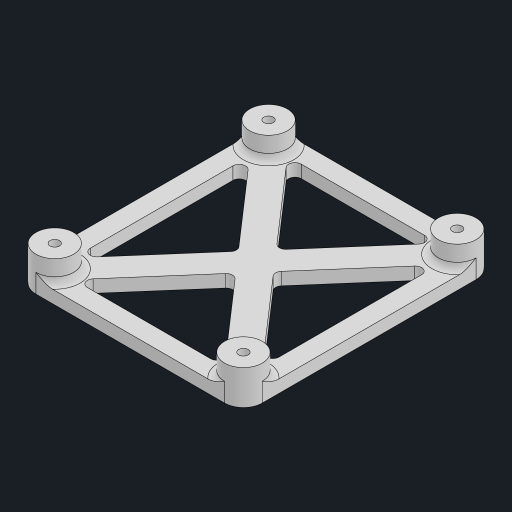
# Autodesk Inventor part: kibanHolder
Saved by Autodesk Inventor 2023 (Build 270158000, 158)
## iProperties
Created: 2022-07-14
Part Number: kibanHolder
Material: 一般
Document SubType Name: Modeling
Designer: legot
Density: 1 g/cm^3
Appearance: 既定
Author: legot
Autodesk Inventor part; units mm, degrees
ref_plane "YZ Plane" through (0, 0, 0) normal (1, 0, 0) x (0, 1, 0)
ref_plane "XZ Plane" through (0, 0, 0) normal (0, 1, 0) x (-1, 0, 0)
ref_plane "XY Plane" through (0, 0, 0) normal (0, 0, 1) x (1, 0, 0)
sketch "スケッチ1" plane through (0, 0, 0) normal (0, 1, 0) x (-1, 0, 0)
  line L0 (15, 17) -> (-15, 17) construction
  line L1 (-15, 17) -> (-15, -17) construction
  line L2 (-15, -17) -> (15, -17) construction
  line L3 (15, -17) -> (15, 17) construction
  circle A0 centre (15, 17) radius 3
  circle A1 centre (15, -17) radius 3
  circle A2 centre (-15, 17) radius 3
  circle A3 centre (-15, -17) radius 3
  line L4 (15, 20) -> (-15, 20)
  line L5 (-15, -20) -> (15, -20)
  line L6 (18, 17) -> (18, -17)
  line L7 (-18, 17) -> (-18, -17)
  line L8 (15, -14) -> (15, 14)
  line L9 (12, 17) -> (-12, 17)
  line L10 (-15, 14) -> (-15, -14)
  line L11 (-12, -17) -> (12, -17)
  line L12 (12, 17) -> (-15, -14)
  line L13 (12, -17) -> (-15, 14)
  line L14 (-12, 17) -> (15, -14)
  line L15 (15, 14) -> (-12, -17)
  point P0 (0, 0)
  point P1 (15, 0)
  point P2 (0, 17)
  point P3 (15, 0)
  point P4 (2.8065, 0)
  point P5 (0, 3.2222)
  point P6 (-2.8065, 0)
  point P7 (0, -3.2222)
  dimension "d0" = 30
  dimension "d1" = 34
  dimension "d4" = 6
  dimension "d5" = 40
  constraints: 32 end point, 12 point on circle, 8 point on line, 6 tangent, 5 parallel, 4 centre point, 4 coincident, 3 equal radius, 2 horizontal, 2 horizontal alignment, 2 midpoint, 1 perpendicular, 1 vertical alignment
  measures "d0" distance of L0.start L0.end
  measures "d1" distance of L2.end L0.start
  measures "d4" diameter of A2
  measures "d5" distance of L5.end L4.start
extrude "押し出し1" add sketch "スケッチ1" along normal blind 2 contours A0 | L6 A1 L8 A0 | A0 L9 A2 L4 | L15 L14 L12 A0 | A1 | A2 | A1 L13 L15 L14 | L15 L13 L12 L14 | L5 A3 L11 A1 | L14 L12 L13 A2 | A2 L10 A3 L7 | L15 A3 L12 L13 | A3
sketch "スケッチ2" plane through (0, 2, 0) normal (0, 1, 0) x (1, 0, 0)
  arc A0 (15, -20) -> (18, -17) centre (15, -17) ccw projected
  arc A1 (-18, -17) -> (-15, -20) centre (-15, -17) ccw projected
  arc A2 (-15, 20) -> (-18, 17) centre (-15, 17) ccw projected
  arc A3 (18, 17) -> (15, 20) centre (15, 17) ccw projected
  circle A4 centre (-15, -17) radius 3 projected
  circle A5 centre (15, -17) radius 3 projected
  circle A6 centre (-15, 17) radius 3 projected
  circle A7 centre (15, 17) radius 3 projected
  point P0 (15, 14)
  point P1 (15, -14)
  point P2 (12, -17)
  point P3 (-12, -17)
  point P4 (-15, -14)
  point P5 (-15, 14)
  point P6 (-12, 17)
  point P7 (12, 17)
  point P8 (0, 0)
extrude "押し出し2" add sketch "スケッチ2" along normal blind 3.5
sketch "スケッチ3" plane through (-15, 5.5, 17) normal (0, 1, 0) x (1, 0, 0)
  circle A0 centre (0, 0) radius 3 projected
  circle A1 centre (0, 34) radius 3 projected
  circle A2 centre (30, 34) radius 3 projected
  circle A3 centre (30, 0) radius 3 projected
  point P0 (15, 17)
hole "穴1" at (-15, 5.5, -17) at (-15, 5.5, 17) at (15, 5.5, -17) at (15, 5.5, 17) direction (0, -1, 0) diameter 1.5 end through all
fillet "フィレット1" radius 1 12 edges at (15, 1, -14) (12, 1, -17) (-15, 1, -14) (-12, 1, -17) (-15, 1, 14) (-12, 1, 17) (12, 1, 17) (15, 1, 14) (0, 1, 3.2222) (0, 1, -3.2222) (2.8065, 1, 0) (-2.8065, 1, 0)
fillet "フィレット2" radius 1 4 edges at (-12.8787, 2, 14.8787) (-12.8787, 2, -14.8787) (12.8787, 2, 14.8787) (12.8787, 2, -14.8787)
